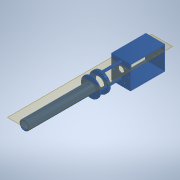
# Autodesk Inventor part: motor bracket
Saved by Autodesk Inventor 2020 (Build 240168000, 168)
## iProperties
Created: 2020-12-24
Part Number: motor bracket
Material: Generic
Document SubType Name: Modeling
Designer: Vikki
Density: 1 g/cm^3
Appearance: Flaked Satin - Blue
Author: Vikki
Autodesk Inventor part; units mm, degrees
ref_plane "YZ Plane" through (0, 0, 0) normal (1, 0, 0) x (0, 1, 0)
ref_plane "XZ Plane" through (0, 0, 0) normal (0, 1, 0) x (-1, 0, 0)
ref_plane "XY Plane" through (0, 0, 0) normal (0, 0, 1) x (1, 0, 0)
sketch "Sketch1" plane through (0, 0, 0) normal (0, 0, 1) x (1, 0, 0)
  circle A0 centre (0, 0) radius 18.5 projected
  arc A1 (-8.9075, 7.6329) -> (8.9075, 7.6329) centre (0, 7) ccw projected
  spline S0 degree 3 poles (8.9075, 7.6329) (8.9044, 7.6769) (8.9082, 7.7215) (8.9387, 7.8037) (8.9677, 7.8415) (9.0503, 7.8747) (9.0975, 7.8677) (9.1766, 7.8302) (9.2105, 7.8009) (9.2388, 7.7672) knots 0 0 0 0 0.25 0.25 0.5 0.5 0.75 0.75 1 1 1 1 projected
  arc A2 (-9.2388, 7.7672) -> (9.2388, 7.7672) centre (0, 0) ccw projected
  spline S1 degree 3 poles (-9.2388, 7.7672) (-9.2105, 7.801) (-9.1766, 7.8302) (-9.0974, 7.8677) (-9.0502, 7.8747) (-8.9678, 7.8415) (-8.9387, 7.8036) (-8.9082, 7.7215) (-8.9044, 7.6769) (-8.9075, 7.6329) knots 0 0 0 0 0.25 0.25 0.5 0.5 0.75 0.75 1 1 1 1 projected
  circle A3 centre (7.75, -13.4234) radius 1.6 projected
  circle A4 centre (-7.75, -13.4234) radius 1.6 projected
  circle A5 centre (-15.5, 0) radius 1.6 projected
  circle A6 centre (-7.75, 13.4234) radius 1.6 projected
  circle A7 centre (7.75, 13.4234) radius 1.6 projected
  circle A8 centre (15.5, 0) radius 1.6 projected
  circle A9 centre (13.4234, 7.75) radius 2.1 projected
  circle A10 centre (-13.4234, 7.75) radius 2.1 projected
  circle A11 centre (0, -15.5) radius 2.1 projected
  circle A12 centre (0, 7) radius 6.25 projected
  line L0 (20, -25) -> (-20, -25)
  line L1 (-20, -25) -> (-20, 25)
  line L2 (-20, 25) -> (20, 25)
  line L3 (20, 25) -> (20, -25)
  line L4 (20, -25) -> (-20, 25) construction
  line L5 (-20, -25) -> (20, 25) construction
  dimension "d0" = 40
  dimension "d1" = 50
  constraints: 12 end point, 2 midpoint, 2 parallel, 1 horizontal, 1 perpendicular
  measures "d0" distance of L1.end L2.end
  measures "d1" distance of L0.end L1.end
extrude "Extrusion1" add sketch "Sketch1" along normal blind 2 contours A0 | A1 S0 A2 S1 | A9 | A10 | A11 | L0 L1 L2 L3
sketch "Sketch2" plane through (0, 0, 2) normal (0, 0, 1) x (1, 0, 0)
  line L0 (-20, -25) -> (20, -25) projected
  line L1 (20, -25) -> (-20, -25)
  line L2 (-20, -25) -> (-20, -27)
  line L3 (-20, -27) -> (20, -27)
  line L4 (20, -27) -> (20, -25)
  line L5 (20, 25) -> (-20, 25) projected
  line L6 (20, 25) -> (-20, 25)
  line L7 (-20, 25) -> (-20, 27)
  line L8 (-20, 27) -> (20, 27)
  line L9 (20, 27) -> (20, 25)
  point P0 (0, 0)
  dimension "d4" = 2
  dimension "d19" = 2
  constraints: 16 end point, 4 parallel, 2 horizontal, 2 perpendicular
  measures "d4" distance of L0.start L2.end
  measures "d19" distance of L5.end L7.end
extrude "Extrusion2" add sketch "Sketch2" against normal blind 70
sketch "Sketch5" plane through (0, 0, -68) normal (0, 0, -1) x (-1, 0, 0)
  line L0 (-20, -27) -> (20, -27)
  line L1 (20, -27) -> (20, 27)
  line L2 (20, 27) -> (-20, 27)
  line L3 (-20, 27) -> (-20, -27)
  circle A0 centre (0, 7) radius 6 construction
  circle A1 centre (0, 7) radius 3 construction
  circle A2 centre (0, 17) radius 1.5
  circle A3 centre (-8.6603, 2) radius 1.5
  circle A4 centre (8.6603, 2) radius 1.5
  point P0 (0, 0)
  dimension "d20" = 10
  dimension "d21" = 3
  dimension "d24" = 360
  constraints: 8 end point, 3 centre point, 2 parallel, 1 horizontal, 1 perpendicular, 1 vertical alignment, 7 other
  measures "d20" distance of A0.centre A2.centre
  measures "d21" diameter of A2
extrude "Extrusion4" add sketch "Sketch5" along normal blind 2
sketch "Sketch6" plane through (0, 0, 2) normal (0, 0, 1) x (1, 0, 0)
  line L0 (20, -27) -> (20, 27) projected
  line L1 (-20, -27) -> (20, -27)
  line L2 (20, -27) -> (20, -20)
  line L3 (20, -20) -> (-20, -20)
  line L4 (-20, -20) -> (-20, -27)
  circle A0 centre (0, 0) radius 18.5 projected
  point P0 (0, 0)
  dimension "d28" = 7
  constraints: 8 end point, 2 parallel, 1 horizontal, 1 perpendicular, 1 point on line
  measures "d28" distance of L1.end L2.end
extrude "Extrusion5" cut sketch "Sketch6" against normal up to surface (72 mm away) contours L1 L4 L3 L0
sketch "Sketch7" plane through (0, 0, 2) normal (0, 0, 1) x (1, 0, 0)
  line L0 (-20, 27) -> (-20, -20) projected
  line L1 (20, -20) -> (20, 27) projected
  line L2 (-20, -20) -> (20, -20)
  line L3 (20, -20) -> (20, -22)
  line L4 (20, -22) -> (-20, -22)
  line L5 (-20, -22) -> (-20, -20)
  point P0 (0, 0)
  dimension "d31" = 2
  constraints: 8 end point, 2 parallel, 1 horizontal, 1 perpendicular
  measures "d31" distance of L1.start L3.end
extrude "Extrusion6" add sketch "Sketch7" against normal up to surface (72 mm away)
sketch "Sketch8" plane through (0, 0, 2) normal (0, 0, 1) x (1, 0, 0)
  circle A0 centre (0, 22) radius 2.5
  circle A1 centre (0, -8) radius 2.5
  point P0 (0, 0)
  dimension "d34" = 22
  dimension "d35" = 5
  dimension "d36" = 8
  constraints: 2 centre point, 2 vertical alignment, 1 equal radius
  measures "d34" distance of point (0, 0) A0.centre
  measures "d35" diameter of A0
  measures "d36" distance of A1.centre point (0, 0)
extrude "Extrusion7" add sketch "Sketch8" along normal blind 46
sketch "Sketch11" plane through (0, 22, 48) normal (0, 0, 1) x (1, 0, 0)
  circle A0 centre (0, -15) radius 8 construction
  circle A1 centre (0, -15) radius 20
  circle A2 centre (0, -15) radius 11
  point P0 (0, -22)
  dimension "d44" = 40
  dimension "d45" = 22
  constraints: 2 centre point, 2 coincident
  measures "d44" diameter of A1
  measures "d45" diameter of A2
extrude "Extrusion9" add sketch "Sketch11" against normal blind 5
sketch "Sketch14" plane through (0, 7, 48) normal (0, 0, 1) x (1, 0, 0)
  circle A0 centre (-15, 0) radius 2
  circle A1 centre (0, 0) radius 6.282 construction
  circle A2 centre (15, 0) radius 2
  point P0 (0, -7)
  dimension "d60" = 15
  dimension "d61" = 4
  dimension "d64" = 360
  constraints: 2 centre point, 1 horizontal alignment, 5 other
  measures "d60" distance of A0.centre A1.centre
  measures "d61" diameter of A0
extrude "Extrusion12" add sketch "Sketch14" along normal blind 15
sketch "Sketch15" plane through (-15, 7, 63) normal (0, 0, 1) x (1, 0, 0)
  circle A0 centre (15, 0) radius 4 construction
  circle A1 centre (15, 0) radius 11 construction
  circle A2 centre (15, 0) radius 20
  circle A3 centre (15, 0) radius 20 projected
  circle A4 centre (15, 0) radius 5
  point P0 (15, -7)
  dimension "d68" = 40
  dimension "d69" = 10
  constraints: 2 centre point, 2 coincident
  measures "d68" diameter of A2
  measures "d69" diameter of A4
extrude "Extrusion13" add sketch "Sketch15" along normal blind 2
sketch "Sketch16" plane through (0, 7, 65) normal (0, 0, 1) x (1, 0, 0)
  circle A0 centre (0, 0) radius 5 construction
  circle A1 centre (0, 0) radius 7.5
  circle A2 centre (0, 0) radius 11 construction
  circle A3 centre (0, 0) radius 10
  point P0 (0, -7)
  dimension "d72" = 15
  dimension "d73" = 20
  constraints: 2 centre point, 2 coincident
  measures "d72" diameter of A1
  measures "d73" diameter of A3
extrude "Extrusion14" add sketch "Sketch16" along normal blind 137.5
ref_plane "Work Plane1" through (0, 17, 65) normal (0, 1, 0) x (-1, 0, 0)
sketch "Sketch17" plane through (0, 17, 65) normal (0, 1, 0) x (-1, 0, 0)
  line L0 (2, 133.5) -> (-2, 133.5)
  line L1 (-2, 133.5) -> (-2, 4)
  line L2 (-2, 4) -> (2, 4)
  line L3 (2, 4) -> (2, 133.5)
  line L4 (-10, 0) -> (-10, 137.5) projected
  line L5 (10, 0) -> (10, 137.5) projected
  line L6 (10, 137.5) -> (-10, 137.5) projected
  line L7 (-10, 0) -> (10, 0) projected
  point P0 (0, -65)
  dimension "d76" = 4
  dimension "d77" = 4
  dimension "d78" = 8
  dimension "d79" = 8
  constraints: 8 end point, 2 parallel, 1 horizontal, 1 perpendicular
  measures "d76" distance between parallel lines of L2 L7
  measures "d77" distance between parallel lines of L6 L0
  measures "d78" distance between parallel lines of L4 L1
  measures "d79" distance between parallel lines of L5 L3
extrude "Extrusion15" cut sketch "Sketch17" against normal up to surface contours L3 L2 L1 L0 round surface about axis through (0, 7, 65) along (0, 0, 1) radius 7.5 far side no
sketch "Sketch18" plane through (0, 0, -70) normal (0, 0, -1) x (-1, 0, 0)
  circle A0 centre (0, 7) radius 6 construction
  circle A1 centre (0, 7) radius 14
  circle A2 centre (0, 17) radius 1.5 projected
  circle A3 centre (-8.6603, 2) radius 1.5 projected
  circle A4 centre (8.6603, 2) radius 1.5 projected
  point P0 (0, 0)
  dimension "d82" = 28
  constraints: 1 centre point, 1 coincident
  measures "d82" diameter of A1
extrude "Extrusion16" add sketch "Sketch18" along normal blind 2.5
sketch "Sketch19" plane through (0, 7, -72.5) normal (0, 0, -1) x (-1, 0, 0)
  circle A0 centre (0, 0) radius 14 construction
  circle A1 centre (0, 0) radius 3.3
  point P0 (0, -7)
  point P1 (-1.4736, 13.9222)
  point P2 (1.4736, 13.9222)
  dimension "d85" = 6.6
  constraints: 1 centre point, 1 coincident
  measures "d85" diameter of A1
extrude "Extrusion17" add sketch "Sketch19" along normal blind 10
body "Solid1"
